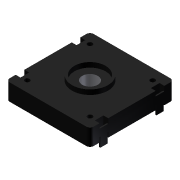
# Autodesk Inventor part: SLIPRING_SRG-1-6G
Saved by Autodesk Inventor 2011 SP1 (Build 150282100, 282)
## iProperties
Created: 2012-05-23
Part Number: SLIPRING_SRG-1-6G
Document SubType Name: Modeling
Designer: arihon
Density: 1 g/cm^3
Author: arihon
Autodesk Inventor part; units mm, degrees
ref_plane "YZ Plane" through (0, 0, 0) normal (1, 0, 0) x (0, 1, 0)
ref_plane "XZ Plane" through (0, 0, 0) normal (0, 1, 0) x (-1, 0, 0)
ref_plane "XY Plane" through (0, 0, 0) normal (0, 0, 1) x (1, 0, 0)
sketch "スケッチ1" plane through (0, 0, 0) normal (0, 0, 1) x (1, 0, 0)
  line L0 (-17.5, 17.5) -> (17.5, 17.5)
  line L1 (17.5, 17.5) -> (17.5, -17.5)
  line L2 (17.5, -17.5) -> (-17.5, -17.5)
  line L3 (-17.5, -17.5) -> (-17.5, 17.5)
  point P0 (0, 0)
  dimension "d0" = 35
  dimension "d1" = 35
  dimension "d2" = 17.5
  dimension "d3" = 17.5
  constraints: 8 end point, 2 parallel, 1 horizontal, 1 perpendicular
  measures "d0" distance of L1.end L2.end
  measures "d1" distance of L2.end L0.start
  measures "d2" distance from line of L2 point (0, 0)
  measures "d3" distance from line of L3 point (0, 0)
extrude "押し出し1" add sketch "スケッチ1" along normal blind 7
sketch "スケッチ2" plane through (0, 0, 7) normal (0, 0, 1) x (1, 0, 0)
  line L0 (-17.5, 17.5) -> (17.5, -17.5)
  line L1 (17.5, 17.5) -> (-17.5, -17.5)
  line L2 (-17.5, -17.5) -> (-17.5, 17.5) projected
  circle A0 centre (0, 0) radius 18.5
  point P0 (-13.0815, 13.0815)
  point P1 (13.0815, 13.0815)
  point P2 (13.0815, -13.0815)
  point P3 (-13.0815, -13.0815)
  dimension "d6" = 37
  constraints: 5 point on line, 4 end point, 4 point on circle, 1 centre point, 1 coincident, 1 perpendicular
  measures "d6" diameter of A0
hole "Hole1" at (-13.0815, 13.0815, 7) at (13.0815, 13.0815, 7) at (13.0815, -13.0815, 7) at (-13.0815, -13.0815, 7) direction (0, 0, -1) diameter 2 end through all
sketch "スケッチ3" plane through (0, 0, 7) normal (0, 0, 1) x (1, 0, 0)
  circle A0 centre (0, 0) radius 7.5
  circle A1 centre (0, 0) radius 6.5
  dimension "d14" = 15
  dimension "d15" = 13
  constraints: 2 centre point, 2 coincident
  measures "d14" diameter of A0
  measures "d15" diameter of A1
extrude "押し出し2" add sketch "スケッチ3" along normal blind 2
sketch "スケッチ4" plane through (0, 0, 7) normal (0, 0, 1) x (1, 0, 0)
  line L0 (17.5, 17.5) -> (17.5, -17.5) projected
  line L1 (-17.5, 17.5) -> (17.5, 17.5) projected
  line L2 (-17.5, -17.5) -> (-17.5, 17.5) projected
  line L3 (17.5, -17.5) -> (-17.5, -17.5) projected
  line L4 (17.5, 13.5) -> (15.5, 13.5)
  line L5 (15.5, 13.5) -> (15.5, 9.9)
  line L6 (15.5, 9.9) -> (17.5, 9.9)
  line L7 (17.5, 9.9) -> (17.5, 13.5)
  line L8 (17.5, 0) -> (-17.5, 0)
  line L9 (17.5, -17.5) -> (17.5, 17.5)
  line L10 (17.5, -13.5) -> (15.5, -13.5)
  line L11 (15.5, -13.5) -> (15.5, -9.9)
  line L12 (15.5, -9.9) -> (17.5, -9.9)
  line L13 (17.5, -9.9) -> (17.5, -13.5)
  line L14 (0, 17.5) -> (0, -17.5)
  line L15 (-17.5, 17.5) -> (-17.5, -17.5)
  line L16 (-17.5, 13.5) -> (-15.5, 13.5)
  line L17 (-15.5, 13.5) -> (-15.5, 9.9)
  line L18 (-15.5, 9.9) -> (-17.5, 9.9)
  line L19 (-17.5, 9.9) -> (-17.5, 13.5)
  line L20 (-17.5, -17.5) -> (-17.5, 17.5)
  line L21 (-15.5, -13.5) -> (-15.5, -9.9)
  line L22 (-15.5, -9.9) -> (-17.5, -9.9)
  line L23 (-17.5, -9.9) -> (-17.5, -13.5)
  line L24 (-17.5, -13.5) -> (-15.5, -13.5)
  dimension "d18" = 4
  dimension "d19" = 2
  dimension "d20" = 3.6
  constraints: 42 end point, 18 symmetric about line, 4 midpoint, 4 point on line, 2 parallel, 1 horizontal, 1 perpendicular
  measures "d18" distance between parallel lines of L1 L4
  measures "d19" distance of L4.start L4.end
  measures "d20" distance of L4.end L5.end
extrude "押し出し3" cut sketch "スケッチ4" against normal blind 2 contours L0 L6 L5 L4 | L16 L17 L18 L2 | L0 L10 L11 L12 | L22 L21 L24 L2
sketch "スケッチ5" plane through (0, 0, 0) normal (0, 0, -1) x (-1, 0, 0)
  line L0 (17.5, 17.5) -> (-17.5, 17.5) projected
  line L1 (-17.5, 17.5) -> (-17.5, -17.5) projected
  line L2 (-17.5, -17.5) -> (17.5, -17.5) projected
  line L3 (17.5, 0) -> (-17.5, 0)
  line L4 (17.5, 17.5) -> (-17.5, 17.5) projected
  line L5 (0, 17.5) -> (0, -17.5)
  line L6 (15.5, 13.5) -> (17, 13.5)
  line L7 (17, 13.5) -> (17, 9.9)
  line L8 (17, 9.9) -> (15.5, 9.9)
  line L9 (15.5, 9.9) -> (15.5, 13.5)
  line L10 (17.5, -17.5) -> (17.5, 17.5) projected
  line L11 (15.5, -13.5) -> (17, -13.5)
  line L12 (17, -13.5) -> (17, -9.9)
  line L13 (17, -9.9) -> (15.5, -9.9)
  line L14 (15.5, -9.9) -> (15.5, -13.5)
  line L15 (-15.5, 13.5) -> (-17, 13.5)
  line L16 (-17, 13.5) -> (-17, 9.9)
  line L17 (-17, 9.9) -> (-15.5, 9.9)
  line L18 (-15.5, 9.9) -> (-15.5, 13.5)
  line L19 (-15.5, -13.5) -> (-17, -13.5)
  line L20 (-17, -13.5) -> (-17, -9.9)
  line L21 (-17, -9.9) -> (-15.5, -9.9)
  line L22 (-15.5, -9.9) -> (-15.5, -13.5)
  line L23 (17, 13.5) -> (15.5, 13.5)
  line L24 (15.5, 13.5) -> (15.5, 9.9)
  line L25 (15.5, 9.9) -> (17, 9.9)
  line L26 (17, 9.9) -> (17, 13.5)
  point P0 (0, 0)
  dimension "d26" = 4
  dimension "d27" = 3.6
  dimension "d28" = 2
  dimension "d29" = 1.5
  constraints: 44 end point, 12 symmetric about line, 4 parallel, 3 midpoint, 2 horizontal, 2 perpendicular
  measures "d26" distance between parallel lines of L0 L6
  measures "d27" distance of L6.end L7.end
  measures "d28" distance between parallel lines of L9 L10
  measures "d29" distance of L6.start L6.end
extrude "押し出し4" cut sketch "スケッチ5" against normal through all contours L6 L7 L8 L9 | L14 L13 L12 L11 | L18 L17 L16 L15 | L19 L20 L21 L22
sketch "スケッチ6" plane through (-17.5, -17.5, 0) normal (-1, 0, 0) x (0, 0, 1)
  line L0 (0, 0) -> (0, 35) projected
  line L1 (0, 35) -> (0, 0) projected
  line L2 (2, 31) -> (0, 31)
  line L3 (0, 31) -> (0, 30.7)
  line L4 (0, 30.7) -> (2, 30.7)
  line L5 (2, 30.7) -> (2, 31)
  line L6 (2, 27.4) -> (0, 27.4)
  line L7 (0, 27.4) -> (0, 27.7)
  line L8 (0, 27.7) -> (2, 27.7)
  line L9 (2, 27.7) -> (2, 27.4)
  line L10 (7, 27.4) -> (7, 7.6) projected
  line L11 (7, 17.5) -> (0, 17.5)
  line L12 (0, 0) -> (0, 35)
  line L13 (2, 4) -> (0, 4)
  line L14 (0, 4) -> (0, 4.3)
  line L15 (0, 4.3) -> (2, 4.3)
  line L16 (2, 4.3) -> (2, 4)
  line L17 (2, 7.6) -> (0, 7.6)
  line L18 (0, 7.6) -> (0, 7.3)
  line L19 (0, 7.3) -> (2, 7.3)
  line L20 (2, 7.3) -> (2, 7.6)
  dimension "d32" = 3
  dimension "d33" = 0.3
  dimension "d34" = 2
  constraints: 36 end point, 10 symmetric about line, 4 parallel, 4 point on line, 3 perpendicular, 2 horizontal, 1 midpoint
  measures "d32" distance between parallel lines of L4 L8
  measures "d33" distance of L8.end L6.start
  measures "d34" distance of L6.start L6.end
extrude "押し出し5" cut sketch "スケッチ6" against normal blind 2
sketch "スケッチ7" plane through (17.5, -17.5, 0) normal (1, 0, 0) x (0, 0, -1)
  line L0 (-7, 27.4) -> (-7, 7.6) projected
  line L1 (-7, 17.5) -> (0, 17.5)
  line L2 (-2, 4.3) -> (0, 4.3)
  line L3 (0, 4.3) -> (0, 4)
  line L4 (0, 4) -> (-2, 4)
  line L5 (-2, 4) -> (-2, 4.3)
  line L6 (-2, 27.4) -> (0, 27.4)
  line L7 (0, 27.4) -> (0, 27.7)
  line L8 (0, 27.7) -> (-2, 27.7)
  line L9 (-2, 27.7) -> (-2, 27.4)
  line L10 (-2, 31) -> (0, 31)
  line L11 (0, 31) -> (0, 30.7)
  line L12 (0, 30.7) -> (-2, 30.7)
  line L13 (-2, 30.7) -> (-2, 31)
  line L14 (0, 7.6) -> (-2, 7.6)
  line L15 (-2, 7.6) -> (-2, 7.3)
  line L16 (-2, 7.3) -> (0, 7.3)
  line L17 (0, 7.3) -> (0, 7.6)
  dimension "d40" = 0.3
  constraints: 34 end point, 8 parallel, 4 horizontal, 4 perpendicular, 1 midpoint
  measures "d40" distance of L4.end L2.start
extrude "押し出し6" cut sketch "スケッチ7" against normal blind 2
sketch "スケッチ8" plane through (0, 0, 0) normal (0, 0, -1) x (-1, 0, 0)
  line L0 (-17, 13.2) -> (-17.5, 13.2) projected
  line L1 (-17.5, 13.2) -> (-17.5, 10.2) projected
  line L2 (-17.5, 10.2) -> (-17, 10.2) projected
  line L3 (-17, 10.2) -> (-17, 13.2) projected
  point P0 (0, 0)
extrude "押し出し7" add sketch "スケッチ8" along normal blind 2
sketch "スケッチ9" plane through (0, 0, 0) normal (0, 0, -1) x (-1, 0, 0)
  line L0 (-17, -10.2) -> (-17.5, -10.2) projected
  line L1 (-17.5, -10.2) -> (-17.5, -13.2) projected
  line L2 (-17.5, -13.2) -> (-17, -13.2) projected
  line L3 (-17, -13.2) -> (-17, -10.2) projected
  point P0 (0, 0)
extrude "押し出し8" add sketch "スケッチ9" along normal blind 2
sketch "スケッチ10" plane through (0, 0, 0) normal (0, 0, -1) x (-1, 0, 0)
  line L0 (17, -13.2) -> (17.5, -13.2) projected
  line L1 (17.5, -13.2) -> (17.5, -10.2) projected
  line L2 (17.5, -10.2) -> (17, -10.2) projected
  line L3 (17, -10.2) -> (17, -13.2) projected
  point P0 (0, 0)
extrude "押し出し9" add sketch "スケッチ10" along normal blind 2
sketch "スケッチ11" plane through (0, 0, 0) normal (0, 0, -1) x (-1, 0, 0)
  line L0 (17.5, 13.2) -> (17, 13.2) projected
  line L1 (17, 13.2) -> (17, 10.2) projected
  line L2 (17, 10.2) -> (17.5, 10.2) projected
  line L3 (17.5, 10.2) -> (17.5, 13.2) projected
  point P0 (0, 0)
extrude "押し出し10" add sketch "スケッチ11" along normal blind 2
fillet "フィレット2" radius 1.5 4 edges at (17.5, -17.5, 3.5) (-17.5, -17.5, 3.5) (-17.5, 17.5, 3.5) (17.5, 17.5, 3.5)
sketch "スケッチ14" plane through (0, 0, 7) normal (0, 0, 1) x (1, 0, 0)
  circle A0 centre (0, 0) radius 6.5 projected
  constraints: 1 coincident
hole "Hole3" at (0, 0, 7) direction (0, 0, -1) diameter 6.5 end through all
equation "\"d1\" = d0"
equation "\"d2\" = 0.5 * d0"
equation "\"d3\" = d2"
